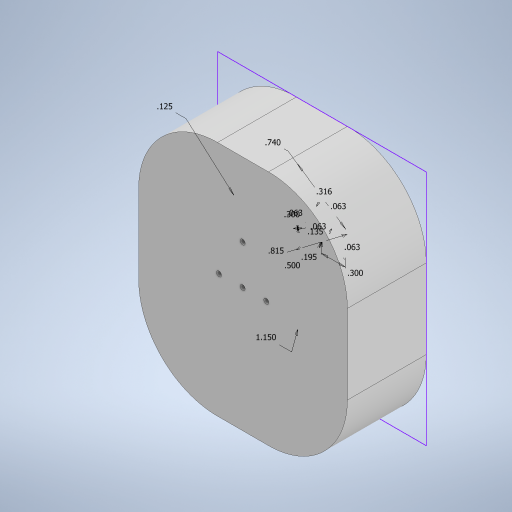
# Autodesk Inventor part: C.Crank on Crankshaft Cutting Jig
Saved by Autodesk Inventor 2023 (Build 270158000, 158)
## iProperties
Created: 2022-10-29
Part Number: C.Crank on Crankshaft Cutting Jig
Material: Generic
Document SubType Name: Modeling
Designer: tommy
Density: 1 g/cm^3
Appearance: Default
Author: tommy
## iProperties of the stored document Crank on Crankshaft_3DPrint.ipt
Created: 2022-10-29
Part Number: Crank on Crankshaft_3DPrint
Material: Generic
Document SubType Name: Modeling
Designer: tommy
Density: 1 g/cm^3
Appearance: Default
Author: tommy
Autodesk Inventor part; units mm, degrees
ref_plane "YZ Plane" through (0, 0, 0) normal (1, 0, 0) x (0, 1, 0)
ref_plane "XZ Plane" through (0, 0, 0) normal (0, 1, 0) x (-1, 0, 0)
ref_plane "XY Plane" through (0, 0, 0) normal (0, 0, 1) x (1, 0, 0)
sketch "Sketch1" plane through (0, 0, 0) normal (0, 0, 1) x (1, 0, 0)
  circle A0 centre (0, 12.7) radius 4.0132
  circle A1 centre (-7.62, 0) radius 1.7145
  circle A2 centre (7.62, 0) radius 1.7145
  circle A3 centre (0, 0) radius 9.525
  arc A4 (-28.992, -3.5622) -> (28.992, -3.5622) centre (0, 0) ccw
  line L0 (-16.51, 12.7) -> (-16.51, 3.175)
  line L1 (16.51, 12.7) -> (16.51, 3.175)
  line L2 (19.685, 0) -> (25.8407, 0)
  line L3 (-19.685, 0) -> (-25.8407, 0)
  arc A5 (16.51, 12.7) -> (-16.51, 12.7) centre (0, 12.7) ccw
  arc A6 (-25.8407, 0) -> (-28.992, -3.5622) centre (-25.8407, -3.175) ccw
  arc A7 (-19.685, 0) -> (-16.51, 3.175) centre (-19.685, 3.175) ccw
  arc A8 (16.51, 3.175) -> (19.685, 0) centre (19.685, 3.175) ccw
  arc A9 (28.992, -3.5622) -> (25.8407, 0) centre (25.8407, -3.175) ccw
  circle A10 centre (0, 12.7) radius 9.398
  circle A11 centre (0, 0) radius 2.4765
  circle A12 centre (0, 0) radius 6.35
  line L4 (-33.494, 36.419) -> (33.7251, 36.419)
  line L5 (33.7251, 36.419) -> (33.7251, -39.9461)
  line L6 (33.7251, -39.9461) -> (-33.494, -39.9461)
  line L7 (-33.494, -39.9461) -> (-33.494, 36.419)
  circle A13 centre (0, 0) radius 10.3505
  circle A14 centre (-7.62, 0) radius 0.7937
  circle A15 centre (0, 0) radius 0.7937
  circle A16 centre (7.62, 0) radius 0.7937
  circle A17 centre (0, 12.7) radius 0.7937
  line L8 (-16.8374, 12.7) -> (-16.8374, 3.175)
  arc A18 (-19.685, 0.3274) -> (-16.8374, 3.175) centre (-19.685, 3.175) ccw
  line L9 (-19.685, 0.3274) -> (-25.8407, 0.3274)
  arc A19 (-25.8407, 0.3274) -> (-29.3169, -3.6021) centre (-25.8407, -3.175) ccw
  arc A20 (-29.3169, -3.6021) -> (29.3169, -3.6021) centre (0, 0) ccw
  arc A21 (29.3169, -3.6021) -> (25.8407, 0.3274) centre (25.8407, -3.175) ccw
  line L10 (25.8407, 0.3274) -> (19.685, 0.3274)
  arc A22 (16.8374, 3.175) -> (19.685, 0.3274) centre (19.685, 3.175) ccw
  line L11 (16.8374, 3.175) -> (16.8374, 12.7)
  arc A23 (16.8374, 12.7) -> (-16.8374, 12.7) centre (0, 12.7) ccw
  point P0 (-16.51, -24.0966)
  point P1 (16.51, -24.0966)
  point P2 (-29.21, 0)
  point P3 (29.21, 0)
  point P4 (-2.1125, 9.2878)
  point P5 (2.1125, 9.2878)
  point P6 (7.0137, 6.4446)
  point P7 (-7.0137, 6.4446)
  point P8 (-6.263, 1.0478)
  point P9 (-6.263, -1.0478)
  point P10 (6.263, -1.0478)
  point P11 (6.263, 1.0478)
  point P12 (4.5198, 4.4602)
  point P13 (-4.5198, 4.4602)
  point P14 (-7.5403, 7.0906)
  point P15 (7.5403, 7.0906)
  dimension "d20" = 8.0264
  dimension "d44" = 3.175
  dimension "d57" = 18.796
  dimension "d70" = 3.429
  dimension "d73" = 29.21
  dimension "d76" = 7.62
  dimension "d77" = 7.62
  dimension "d84" = 12.7
  dimension "d85" = 4.953
  dimension "d97" = 1.5875
  dimension "d98" = 1.5875
  dimension "d99" = 1.5875
  dimension "d100" = 1.5875
  dimension "d109" = 20.701
  constraints: 28 point on circle, 24 centre point, 24 end point, 8 coincident, 8 tangent, 4 equal radius, 4 point on line, 3 horizontal, 2 parallel, 2 vertical, 1 perpendicular, 9 other
  measures "d20" diameter of A0
  measures "d44" radius of A6
  measures "d57" diameter of A10
  measures "d70" diameter of A1
  measures "d73" radius of A4
  measures "d76" distance of A3.centre A2.centre
  measures "d77" distance of A3.centre A1.centre
  measures "d84" diameter of A12
  measures "d85" diameter of A11
  measures "d97" diameter of A14
  measures "d98" diameter of A15
  measures "d99" diameter of A16
  measures "d100" diameter of A17
  measures "d109" diameter of A13
extrude "Extrusion22" add sketch "Sketch1" along normal blind 25.4 contours A0 A13 | A0 A13 A10 | A13 A0 A3 | A0 A3 A10 A13 | A13 A10 A3 A0 | A3 A0 | A0 A3 A10 A12 | A10 A3 A13 | A10 A12 A1 A2 A3 | A12 A10 | A10 A12 A2 A1 | A12 A1 | A1 A12 | A12 A2 | A2 A12 | A6 L3 A7 L0 A5 L1 A8 L2 A9 A4 | A11 | L4 L5 L6 L7 | A23 L11 A22 L10 A21 A20 A19 L9 A18 L8
extrude "Extrusion23" cut sketch "Sketch1" along normal blind 19.304 contours A10 A3 A13 | A10 A12 A1 A2 A3 | A10 A12 A2 A1 | A12 A1 | A1 A12 | A12 A2 | A2 A12 | A11 | A14 | A15 | A16
extrude "Extrusion24" cut sketch "Sketch1" along normal blind 11.43 contours A0 A13 | A0 A13 A10 | A13 A0 A3 | A0 A3 A10 A13 | A13 A10 A3 A0 | A3 A0 | A0 A3 A10 A12 | A10 A3 A13 | A10 A12 A1 A2 A3 | A12 A10 | A10 A12 A2 A1 | A12 A1 | A1 A12 | A12 A2 | A2 A12 | A6 L3 A7 L0 A5 L1 A8 L2 A9 A4 | A11 | A14 | A15 | A16 | A17
fillet "Fillet4" radius 1.016 1 edges at (0, -10.3505, 11.43)
fillet "Fillet5" radius 25.4 4 edges at (33.7251, -39.9461, 12.7) (-33.494, -39.9461, 12.7) (-33.494, 36.419, 12.7) (33.7251, 36.419, 12.7)
body "Solid5"
